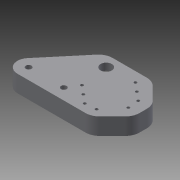
# Autodesk Inventor part: joint1left+ax12imprint_v3
Saved by Autodesk Inventor 2014 (Build 180170000, 170)
## iProperties
Created: 2014-01-16
Part Number: joint1left+ax12imprint_v3
Material: Générique
Document SubType Name: Modeling
Designer: helly
Density: 1 g/cm^3
Appearance: Par défaut
Author: helly
Autodesk Inventor part; units mm, degrees
ref_plane "YZ Plane" through (0, 0, 0) normal (1, 0, 0) x (0, 1, 0)
ref_plane "XZ Plane" through (0, 0, 0) normal (0, 1, 0) x (-1, 0, 0)
ref_plane "XY Plane" through (0, 0, 0) normal (0, 0, 1) x (1, 0, 0)
sketch "Esquisse1" plane through (0, 0, 0) normal (0, 0, 1) x (1, 0, 0)
  circle A0 centre (0, 0) radius 2
  line L0 (0, 0) -> (46.5696, 0) construction
  line L1 (0, 0) -> (27.5772, 27.5772) construction
  circle A1 centre (27.5772, 27.5772) radius 2
  line L2 (27.5772, 27.5772) -> (55.1548, 4.4368) construction
  line L3 (27.5772, 27.5772) -> (45.4581, 27.5772) construction
  line L4 (0, 0) -> (0, -8) construction
  line L5 (0, 0) -> (-5.6569, 5.6569) construction
  line L6 (27.5772, 27.5772) -> (27.5772, 35.5772) construction
  line L7 (27.5772, 27.5772) -> (36.2548, 37.9188) construction
  line L8 (36.2548, 37.9188) -> (41.2341, 33.7406) construction
  line L9 (41.2341, 33.7406) -> (47.3624, 28.5983) construction
  line L10 (47.3624, 28.5983) -> (53.4908, 23.456) construction
  line L11 (53.4908, 23.456) -> (59.6192, 18.3137) construction
  line L12 (55.1548, 4.4368) -> (60.2971, 10.5652) construction
  circle A2 centre (41.2341, 33.7406) radius 1 construction
  circle A3 centre (47.3624, 28.5983) radius 1
  circle A4 centre (53.4908, 23.456) radius 1
  circle A5 centre (59.6192, 18.3137) radius 1
  circle A6 centre (60.2971, 10.5652) radius 1
  line L13 (59.6192, 18.3137) -> (67.6192, 18.3137) construction
  line L14 (67.6192, 35.5772) -> (67.6192, -8)
  line L15 (67.6192, -8) -> (-17.1163, -8)
  line L16 (-17.1163, -8) -> (19.4493, 35.5772)
  line L17 (19.4493, 35.5772) -> (67.6192, 35.5772)
  circle A7 centre (23.8788, 13.0574) radius 1 construction
  circle A8 centre (30.0072, 7.9151) radius 1
  circle A9 centre (36.1355, 2.7728) radius 1
  circle A10 centre (42.2639, -2.3695) radius 1
  circle A11 centre (50.0125, -1.6915) radius 1
  line L18 (0, 0) -> (25, 0) construction
  circle A12 centre (25, 0) radius 2
  dimension "d0" = 4
  dimension "d1" = 39
  dimension "d2" = 45
  dimension "d3" = 36
  dimension "d4" = 40
  dimension "d5" = 8
  dimension "d6" = 8
  dimension "d7" = 8
  dimension "d8" = 13.5
  dimension "d9" = 6.5
  dimension "d10" = 8
  dimension "d11" = 8
  dimension "d12" = 8
  dimension "d13" = 8
  dimension "d14" = 2
  dimension "d15" = 8
  dimension "d16" = 25
  constraints: 38 end point, 13 centre point, 8 coincident, 8 perpendicular, 6 equal radius, 5 point on line, 5 symmetric about line, 4 parallel, 3 collinear, 1 horizontal, 5 other
  measures "d0" diameter of A0
  measures "d1" distance of L0.start L1.end
  measures "d2" angle of L0 L1
  measures "d3" distance of L2.start L2.end
  measures "d4" angle of L2 L3
  measures "d5" distance of L0.start L4.end
  measures "d6" distance of L0.start L5.end
  measures "d7" distance of L2.start L6.end
  measures "d8" distance of L2.start L7.end
  measures "d9" distance of L7.end L8.end
  measures "d10" distance of L8.end L9.end
  measures "d11" distance of L9.end L10.end
  measures "d12" distance of L10.end L11.end
  measures "d13" distance of L2.end L12.end
  measures "d14" diameter of A2
  measures "d15" distance of L13.start L13.end
  measures "d16" distance of L0.start L18.end
extrude "Extrusion1" add sketch "Esquisse1" along normal blind 12
sketch "Esquisse2" plane through (0, 0, 0) normal (0, 0, -1) x (-1, 0, 0)
  circle A0 centre (-27.5772, 27.5772) radius 2 projected
  circle A1 centre (0, 0) radius 2 projected
  line L0 (17.1163, -8) -> (-19.4493, 35.5772) projected
  line L1 (-19.4493, 35.5772) -> (-67.6192, 35.5772) projected
  circle A2 centre (-27.5772, 27.5772) radius 12 construction
  line L2 (-39.5772, 35.5772) -> (-39.5772, 27.5772)
  line L3 (4.7219, 6.771) -> (-30.5997, 15.964)
  arc A3 (-39.5772, 27.5772) -> (-30.5997, 15.964) centre (-27.5772, 27.5772) ccw
  line L4 (-67.6192, -8) -> (17.1163, -8) projected
  line L5 (0, 0) -> (0, 8) construction
  dimension "d19" = 24
  dimension "d42" = 8
  constraints: 6 end point, 4 point on circle, 3 point on line, 2 centre point, 2 coincident, 2 perpendicular, 2 tangent
  measures "d19" diameter of A2
  measures "d42" distance of L5.start L5.end
extrude "Extrusion2" cut sketch "Esquisse2" against normal blind 7 contours L3 A3 L2 L1 L0
sketch "Esquisse3" plane through (0, 0, 7) normal (0, 0, -1) x (-1, 0, 0)
  circle A0 centre (-27.5772, 27.5772) radius 2 projected
  arc A1 (-39.5772, 27.5772) -> (-30.5997, 15.964) centre (-27.5772, 27.5772) ccw projected
  circle A2 centre (-27.5772, 27.5772) radius 4
  point P0 (0, 0)
  dimension "d24" = 8
  constraints: 1 centre point, 1 coincident
  measures "d24" diameter of A2
extrude "Extrusion3" cut sketch "Esquisse3" against normal through all
fillet "Congé1" radius 8 1 edges at (-17.1163, -8, 6)
fillet "Congé2" radius 10 1 edges at (19.4493, 35.5772, 9.5)
fillet "Congé5" radius 8 1 edges at (39.5772, 35.5772, 3.5)
chamfer "Chanfrein1" distance 15 angle 45 1 edges at (67.6192, 35.5772, 6)
chamfer "Chanfrein2" distance 15 angle 45 1 edges at (67.6192, -8, 6)
fillet "Congé6" radius 10 1 edges at (67.6192, 20.5772, 6)
fillet "Congé7" radius 10 1 edges at (52.6192, 35.5772, 6)
fillet "Congé8" radius 10 1 edges at (67.6192, 7, 6)
fillet "Congé9" radius 10 1 edges at (52.6192, -8, 6)
